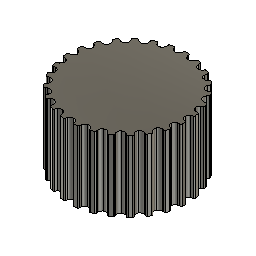
gear_27z (Autodesk Fusion 360 design; units mm, degrees)
Autodesk Fusion 360 part; units mm, degrees
sketch "Sketch1" plane through (0, 0, 0) normal (0, 0, 1) x (1, 0, 0) in component "gt2 pulley"
  circle A0 centre (0, 0) radius 8.5944 construction
  circle A1 centre (0, 0) radius 7.5904 construction
  line L0 (0, 0) -> (0, 8.5944) construction
  line L1 (0, 0) -> (0.9977, 8.5363) construction
  line L2 (0, 0) -> (1.4107, 8.4778) construction
  circle A2 centre (0, 0) radius 8.3404 construction
  arc A3 (0.3696, 8.1926) -> (0.4176, 7.9195) centre (1.369, 8.2272) ccw
  circle A4 centre (0, 0) radius 8.1904 construction
  arc A5 (0.2237, 8.3374) -> (0, 8.3404) centre (0, 0) ccw
  arc A6 (0.3696, 8.1926) -> (0.2237, 8.3374) centre (0.2197, 8.1874) ccw
  arc A7 (0.4176, 7.9195) -> (0.8812, 7.539) centre (0.9456, 8.0903) ccw
  arc A8 (0, 8.3404) -> (-0.2237, 8.3374) centre (0, 0) ccw
  arc A9 (-0.2237, 8.3374) -> (-0.3696, 8.1926) centre (-0.2197, 8.1874) ccw
  arc A10 (-0.4176, 7.9195) -> (-0.3696, 8.1926) centre (-1.369, 8.2272) ccw
  arc A11 (-0.8812, 7.539) -> (-0.4176, 7.9195) centre (-0.9456, 8.0903) ccw
  arc A12 (0.8812, 7.539) -> (-0.8812, 7.539) centre (0, 0) ccw
  point P0 (1.369, 8.2272)
  point P1 (0, 8.3404)
  dimension "d18" = 17.1887
  dimension "d19" = 6.667
  dimension "d22" = 1.004
  dimension "d24" = 0.75
  dimension "d26" = 1
  dimension "d27" = 0.15
  dimension "d28" = 0.15
  dimension "d47" = 0.555
  dimension "d52" = 3.812
  constraint coincident A0.centre A1.centre
  constraint coincident A0 L0.end
  constraint vertical L0
  constraint coincident A0 L1.end
  constraint coincident A0 L2.end
  constraint concentric A1 A2
  constraint coincident A1 A7.end
  constraint coincident L1 A7.end
  constraint coincident A2 P0
  constraint coincident L2 P0
  constraint coincident P0 A3.centre
  constraint coincident A2 P1
  constraint coincident L0 P1
  constraint concentric A2 A4
  constraint coincident P1 A5.end
  constraint coincident A4 A6.centre
  constraint coincident A3.start A6.start
  constraint tangent A3 A6
  constraint tangent A3 A7
  constraint symmetric L0 A7.end A11.start
  constraint symmetric L0 A3.start A9.end
  constraint symmetric L0 A3.end A10.start
  constraint symmetric L0 A3 A10
  constraint symmetric L0 A5.start A8.end
  constraint symmetric L0 P1 A5.end
  constraint symmetric L0 A5 A8
  constraint symmetric L0 A6 A9
  constraint symmetric L0 A7 A11
  constraint coincident A1 A11.start
  constraint tangent A1 A7
  constraint coincident L1 A7.centre
  measures "d18" diameter of A0
  measures "d19" angle of L0 L1
  measures "d22" distance of A0 A1
  measures "d24" distance of A1 A2
  measures "d26" radius of A3
  measures "d27" distance of A2 A4
  measures "d28" radius of A6
  measures "d47" radius of A7
extrude "Extrude1" add sketch "Sketch1" along normal blind 10 makes body 1
pattern_circular "C-Pattern1" count 27 over 360 about axis through (0, 0, 1.75) along (0, 0, 1) of bodies 1 makes body 2 at (-1.8458, 7.3625, 6.6667) makes body 3 at (-4.0056, 6.4474, 6.6667) makes body 4 at (-5.3845, 5.3498, 6.6667) makes body 5 at (-6.1465, 4.4536, 6.6667) makes body 6 at (-7.2128, 2.3642, 6.6667) makes body 7 at (-7.3253, 1.9882, 3.3333) makes body 8 at (-7.5864, 0.2453, 6.6667) makes body 9 at (-7.4385, -1.5109, 3.3333) makes body 10 at (-6.5238, -3.8798, 6.6667) makes body 11 at (-5.9692, -4.6885, 3.3333) makes body 12 at (-4.0886, -6.395, 6.6667) makes body 13 at (-1.9408, -7.338, 6.6667) makes body 14 at (-0.7837, -7.5498, 6.6667) makes body 15 at (0.1962, -7.5878, 3.3333) makes body 16 at (2.688, -7.0985, 6.6667) makes body 17 at (4.727, -5.9388, 6.6667) makes body 18 at (5.0277, -5.6865, 3.3333) makes body 19 at (6.2036, -4.3737, 3.3333) makes body 20 at (7.045, -2.8252, 3.3333) makes body 21 at (7.5826, -0.3433, 6.6667) makes body 22 at (7.4574, 1.4146, 6.6667) makes body 23 at (7.2128, 2.3642, 3.3333) makes body 24 at (5.6539, 5.0643, 6.6667) makes body 25 at (5.3845, 5.3498, 3.3333) makes body 26 at (2.7796, 7.0631, 6.6667) makes body 27 at (2.4108, 7.1973, 3.3333)
sketch "Sketch2" plane through (0, 0, 10) normal (0, 0, 1) x (-1, 0, 0)
  arc A0 (-8.1573, 0.8454) -> (-8.3103, 0.7081) centre (-8.1608, 0.6954) ccw
  arc A1 (-8.3103, 0.7081) -> (-8.3363, 0.2615) centre (0, 0) ccw
  arc A2 (-8.3363, 0.2615) -> (-8.2002, 0.1074) centre (-8.1863, 0.2567) ccw
  arc A3 (-7.9304, 0.0436) -> (-8.2002, 0.1074) centre (-8.2929, -0.8883) ccw
  arc A4 (-7.5775, -0.4413) -> (-7.9304, 0.0436) centre (-8.1316, -0.4736) ccw
  arc A5 (-7.4751, 1.3181) -> (-7.5775, -0.4413) centre (0, 0) ccw
  arc A6 (-7.8818, 0.8773) -> (-7.4751, 1.3181) centre (-8.0216, 1.4144) ccw
  arc A7 (-8.1573, 0.8454) -> (-7.8818, 0.8773) centre (-8.1337, 1.8451) ccw
  circle A8 centre (0, 0) radius 7.5904
  constraint concentric A1 A8
extrude "Extrude2" add sketch "Sketch2" against normal blind 10 contours A5 A8 bodies 1 2 3 4 5 7 8 9 10 11 12 13 14 16 17 19 20 21 22 24 25 27
combine "Combine1" operation add target body 1 tool bodies 26 18 23 6 15
extrude "Extrude4" [suppressed] in component "gt2 pulley"
pattern_circular "C-Pattern7" [suppressed] in component "gt2 pulley"
extrude "Extrude3" [suppressed] in component "gt2 pulley"
pattern_circular "C-Pattern6" [suppressed] in component "gt2 pulley"
extrude "Extrude2'" [suppressed] in component "gt2 pulley"
pattern_circular "C-Pattern5" [suppressed] in component "gt2 pulley"
extrude "Extrude1'" [suppressed] in component "gt2 pulley"
pattern_circular "C-Pattern4" [suppressed] in component "gt2 pulley"
pattern_circular "C-Pattern3" [suppressed] in component "gt2 pulley"
pattern_circular "C-Pattern2" [suppressed] in component "gt2 pulley"
pattern_circular "C-Pattern1'" [suppressed] in component "gt2 pulley"
copy_body "Body->Comp1" [suppressed] in component "Component"
copy_body "Body->Comp2" [suppressed] in component "Component'"
copy_body "Body->Comp3" [suppressed] in component "Component''"
copy_body "Body->Comp4" [suppressed] in component "Component'''"
copy_body "Body->Comp5" [suppressed] in component "Component''''"
copy_body "Body->Comp6" [suppressed] in component "Component'''''"
copy_body "Body->Comp7" [suppressed] in component "Component''''''"
copy_body "Body->Comp8" [suppressed] in component "Component'''''''"
copy_body "Body->Comp9" [suppressed] in component "Component''''''''"
copy_body "Body->Comp10" [suppressed] in component "Component'''''''''"
copy_body "Body->Comp11" [suppressed] in component "Component''''''''''"
copy_body "Body->Comp12" [suppressed] in component "Component'''''''''''"
copy_body "Body->Comp13" [suppressed] in component "Component''''''''''''"
copy_body "Body->Comp14" [suppressed] in component "Component'''''''''''''"
copy_body "Body->Comp15" [suppressed] in component "Component''''''''''''''"
copy_body "Body->Comp16" [suppressed] in component "Component'''''''''''''''"
copy_body "Body->Comp17" [suppressed] in component "Component''''''''''''''''"
copy_body "Body->Comp18" [suppressed] in component "Component'''''''''''''''''"
copy_body "Body->Comp19" [suppressed] in component "Component''''''''''''''''''"
copy_body "Body->Comp20" [suppressed] in component "Component'''''''''''''''''''"
component "gt2 pulley" placed x (1, 0, 0) y (0, 1, 0) z (0, 0, 1) at (0, 0, 0)
equation "NumTeeth = 27" comment "min 20"
equation "ToothPitch = 2 mm"
equation "PullyDia = NumTeeth * ToothPitch / PI"
equation "ToothAng = ( ( 360 / NumTeeth ) * 1 deg )"
equation "TransOffsetAngle = ToothAng * 0.2"
equation "Sholulder_Radius = 0.15 mm"
equation "Root_Radius = 0.555 mm"
equation "TransRadius = 1 mm"
equation "ToolHeight = 0.75 mm"
equation "PLD = 0.254 mm"
equation "d18 = PullyDia"
equation "d19 = ToothAng / 2"
equation "d22 = PLD + ToolHeight"
equation "d24 = ToolHeight"
equation "d26 = TransRadius"
equation "d27 = Sholulder_Radius"
equation "d31 = NumTeeth"
equation "d33 = NumTeeth"
equation "d35 = NumTeeth"
equation "d37 = NumTeeth"
equation "d41 = NumTeeth"
equation "d45 = NumTeeth"
equation "d47 = Root_Radius"
equation "d50 = NumTeeth"
